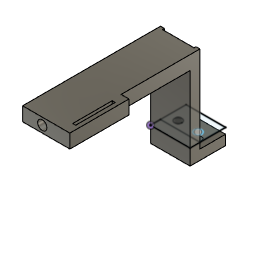
wiperv2 (Autodesk Fusion 360 design; units mm, degrees)
Autodesk Fusion 360 part; units mm, degrees
sketch "Skizze1" plane through (0, 0, 0) normal (0, 0, 1) x (1, 0, 0)
  line L0 (0, 0) -> (20, 0)
  line L1 (20, 0) -> (20, 18)
  line L2 (20, 18) -> (0, 18)
  line L3 (0, 18) -> (0, 0)
  circle A0 centre (15, 9) radius 1.85
  circle A1 centre (5, 9) radius 1.85
  line L4 (0, 0) -> (0, 5)
  line L5 (0, 5) -> (20, 5)
  dimension "d1" = 20
  dimension "d2" = 18
  dimension "d3" = 3.7
  dimension "d4" = 3.7
  dimension "d5" = 5
  constraint horizontal L0
  constraint vertical L1
  constraint horizontal L2
  constraint vertical L3
  constraint coincident L0.start L3.end
  constraint perpendicular L0 L4
  constraint coincident L1 L5.end
  constraint perpendicular L1 L5
  measures "d1" distance of L0.start L0.end
  measures "d2" distance of L0.start L2.end
  measures "d3" diameter of A0
  measures "d4" diameter of A1
  measures "d5" distance of L0.start L4.end
extrude "Extrusion1" add sketch "Skizze1" along normal blind 40 contours L0 L1 L3 L4 L5
extrude "Extrusion2" add sketch "Skizze1" along normal blind 5 contours L1 L2 L3 L5
box "Grundkörper Quader1" add length 5 width 20 height 65 placed x (0, 0, -1) y (1, 0, 0) z (0, -1, 0) at (0, 0, 40)
box "Grundkörper Quader2" cut length 1 width 10 height -35 placed x (0, 0, -1) y (1, 0, 0) z (0, -1, 0) at (5, 0, 35)
extrude "Extrusion3" cut 1 faces at (15, 3.3333, 34.3333) along direction (1, 0, 0) blind 3
extrude "Extrusion4" cut 1 faces at (5, 3.3333, 34.3333) along direction (-1, 0, 0) blind 3
box "Grundkörper Quader3" cut length 5 width 16 height -1 placed x (0, 0, 1) y (1, 0, 0) z (0, 1, 0) at (2, 5, 35)
hole "Bohrung1" at (10, -65, 37.5) direction (0, 1, 0) diameter 4.75 depth 6 tip angle 180
extrude "Extrusion5" add sketch "Skizze1" against normal blind 5
extrude "Extrusion6" cut 1 faces at (8.5586, 15.574, 5) along direction (0, 0, -1) blind 5
extrude "Extrusion7" add 1 faces at (8.5586, 2.426, -5) along direction (0, 0, -1) blind 3
extrude "Extrusion8" cut sketch "Skizze1" against normal blind 3 contours L1 L2 L3 L5
extrude "Extrusion9" add 1 faces at (12.6667, -42, 40) along direction (0, 0, 1) blind 1
extrude "Extrusion10" cut 1 faces at (12.6667, 1.6667, 34) along direction (0, 0, -1) blind 2
extrude "Extrusion11" add 1 faces at (12.6667, -43.3333, 35) along direction (0, 0, -1) blind 1
chamfer "Fase1" distance 4 distance2 2 1 edges at (10, 4, 34) measured on face at (12.6667, -43.3333, 34)
box "Grundkörper Quader4" add length 7 width 30 height 4 placed x (0, 0, 1) y (0, -1, 0) z (1, 0, 0) at (20, -35, 34)
box "Grundkörper Quader5" add length 25 width 2 height 1 placed x (0, -1, 0) y (-1, 0, 0) z (0, 0, -1) at (24, -35, 34)
box "Grundkörper Quader6" cut length 20 width 1.5 height -14 placed x (0, 1, 0) y (1, 0, 0) z (0, 0, -1) at (20.5, -60, 34)
extrude "Extrusion12" cut 1 faces at (22.6667, -43.3333, 33) along direction (0, 0, 1) blind 1
